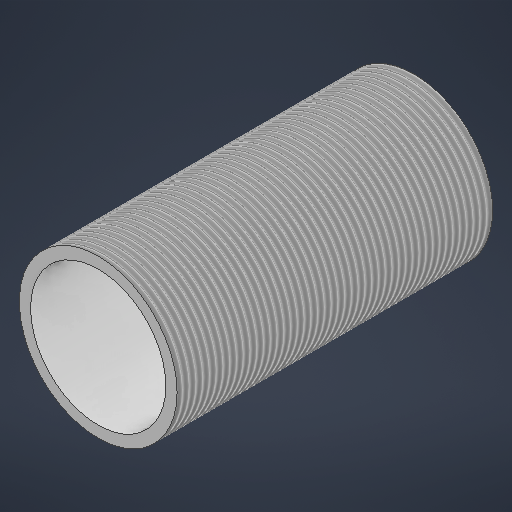
# Autodesk Inventor part: macro-hueco-thread
Saved by Autodesk Inventor 2027 (Build 310192060, 192F)
## iProperties
Created: 2026-06-08
Part Number: macro-hueco-thread
Material: Generic
Document SubType Name: Modeling
Designer: andyv
Density: 1 g/cm^3
Appearance: Default
Author: andyv
Autodesk Inventor part; units mm, degrees
ref_plane "YZ Plane" through (0, 0, 0) normal (1, 0, 0) x (0, 1, 0)
ref_plane "XZ Plane" through (0, 0, 0) normal (0, 1, 0) x (-1, 0, 0)
ref_plane "XY Plane" through (0, 0, 0) normal (0, 0, 1) x (1, 0, 0)
sketch "Sketch1" plane through (0, 0, 0) normal (0, 0, 1) x (1, 0, 0)
  circle A0 centre (0, 0) radius 17.5
  circle A1 centre (0, 0) radius 15
  constraints: 2 centre point
extrude "Extrusion1" add sketch "Sketch1" along normal blind 70 contours A0 | A1
sketch "Sketch2" plane through (0, 0, 0) normal (0, 0, 1) x (1, 0, 0)
  circle A0 centre (0, 0) radius 15
  constraints: 1 centre point
extrude "Extrusion2" cut sketch "Sketch2" along normal blind 70
thread "Thread1" size "M35x1.5" class "6g" standard "ANSI Metric M Profile" full length
body "Solid1"
